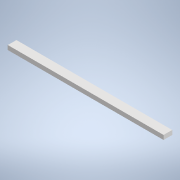
# Autodesk Inventor part: Stock
Saved by Autodesk Inventor 2022 (Build 260153000, 153)
## iProperties
Created: 2022-03-03
Part Number: Stock
Material: Generic
Document SubType Name: Modeling
Designer: Nathan Griffith
Density: 1 g/cm^3
Appearance: Default
Author: Nathan Griffith
Autodesk Inventor part; units mm, degrees
ref_plane "YZ Plane" through (0, 0, 0) normal (1, 0, 0) x (0, 1, 0)
ref_plane "XZ Plane" through (0, 0, 0) normal (0, 1, 0) x (-1, 0, 0)
ref_plane "Work Plane1" through (-455.2, 25.4, 3.7) normal (0, 1, 0) x (0, 0, 1)
sketch "Sketch1" plane through (0, 0, 0) normal (0, 1, 0) x (-1, 0, 0)
  line L0 (0, 0) -> (457.2, 0)
  line L1 (457.2, 0) -> (457.2, 25.4)
  line L2 (457.2, 25.4) -> (0, 25.4)
  line L3 (0, 25.4) -> (0, 0)
  dimension "d0" = 457.2
  dimension "d1" = 25.4
  constraints: 8 end point, 2 parallel, 1 horizontal, 1 perpendicular
  measures "d0" distance of L2.end L1.end
  measures "d1" distance of L1.end L0.end
extrude "Extrusion1" add sketch "Sketch1" against normal blind 12.7 from surface at 25.4
body "Solid1"
